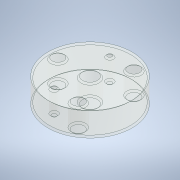
# Autodesk Inventor part: water
Saved by Autodesk Inventor 2020 (Build 240168000, 168)
## iProperties
Created: 2019-06-21
Part Number: water
Material: PAEK Plastic
Document SubType Name: Modeling
Designer: ColinP
Density: 1.32 g/cm^3
Appearance: Clear
Mass: 2.13746 g
Surface Area: 21.7191 cm^2
Volume: 2.13746 cm^3
Author: ColinP
Autodesk Inventor part; units mm, degrees
ref_plane "YZ Plane" through (0, 0, 0) normal (1, 0, 0) x (0, 1, 0)
ref_plane "XZ Plane" through (0, 0, 0) normal (0, 1, 0) x (-1, 0, 0)
ref_plane "XY Plane" through (0, 0, 0) normal (0, 0, 1) x (1, 0, 0)
sketch "Sketch1" plane through (0, 0, 0) normal (0, 1, 0) x (-1, 0, 0)
  circle A0 centre (0, 0) radius 17.78
  dimension "d0" = 35.56
  constraints: 1 centre point, 1 coincident
  measures "d0" diameter of A0
extrude "Extrusion1" add sketch "Sketch1" along normal blind 10.16
sketch "Sketch2" plane through (0, 10.16, 0) normal (0, 1, 0) x (1, 0, 0)
  circle A0 centre (0, 0) radius 17.78 projected
  constraints: 1 coincident
hole "Hole1" at (0, 10.16, 0) direction (0, -1, 0) diameter 6.35 end through all
sketch "Sketch3" plane through (0, 10.16, 0) normal (0, 1, 0) x (1, 0, 0)
  line L0 (0, 0) -> (-13.6144, 0)
  dimension "d10" = 13.6144
  constraints: 2 end point, 1 horizontal
  measures "d10" distance of L0.start L0.end
hole "Hole2" at (-13.6144, 10.16, 0) direction (0, -1, 0) diameter 4.9022 end through all
pattern_circular "Circular Pattern1" count 3 over 360 about axis through (0, -41.1455, 0) along (0, 1, 0) of "Hole2"
sketch "Sketch5" plane through (0, 10.16, 0) normal (0, 1, 0) x (1, 0, 0)
  circle A0 centre (-13.6144, 0) radius 2.4511 projected
  circle A1 centre (6.8072, 11.7904) radius 2.4511 projected
  line L0 (-13.6144, 0) -> (6.8072, 11.7904)
  circle A2 centre (6.8072, -11.7904) radius 2.4511 projected
  line L1 (6.8072, 11.7904) -> (6.8072, -11.7904)
  line L2 (6.8072, -11.7904) -> (-13.6144, 0)
  line L3 (-13.6144, 0) -> (-13.6144, -11.7904)
  line L4 (-13.6144, -11.7904) -> (6.8072, -11.7904)
  line L5 (-13.6144, 0) -> (-13.6144, 11.7904)
  line L6 (-13.6144, 11.7904) -> (6.8072, 11.7904)
  circle A3 centre (-3.4036, 11.7904) radius 0.635
  circle A4 centre (-3.4036, -11.7904) radius 0.635
  point P0 (0, 0)
  dimension "d28" = 1.27
  constraints: 14 end point, 2 centre point, 2 midpoint, 2 vertical, 1 perpendicular, 1 point on line
  measures "d28" diameter of A3
hole "Hole4" at (-3.4036, 10.16, 11.7904) at (-3.4036, 10.16, -11.7904) direction (0, -1, 0) diameter 1.905 end through all
shell "Shell1" thickness 0.635 removed faces 0
body "Solid1"
